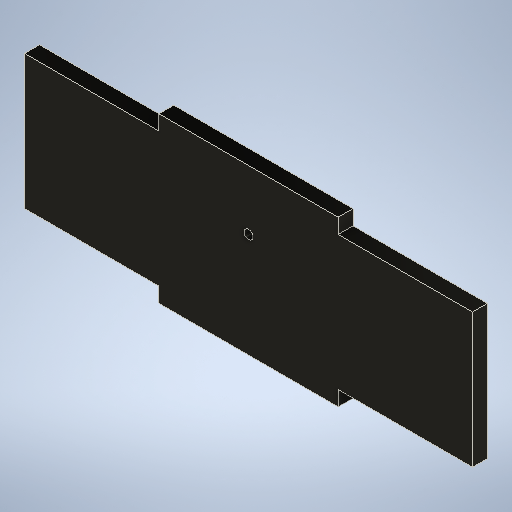
# Autodesk Inventor part: FRONT_1
Saved by Autodesk Inventor 2025.3 (Build 293356030, 356C)
## iProperties
Created: 2026-06-30
Part Number: FRONT_1
Material: ABS Plastic
Document SubType Name: Modeling
Designer: user
Density: 1.06 g/cm^3
Appearance: Gunmetal
Author: user
Autodesk Inventor part; units mm, degrees
ref_plane "YZ Plane" through (0, 0, 0) normal (1, 0, 0) x (0, 1, 0)
ref_plane "XZ Plane" through (0, 0, 0) normal (0, 1, 0) x (-1, 0, 0)
ref_plane "XY Plane" through (0, 0, 0) normal (0, 0, 1) x (1, 0, 0)
sketch "Sketch1" plane through (0, 0, 0) normal (0, 0, 1) x (1, 0, 0)
  line L0 (0, 0) -> (150, 0)
  line L1 (150, 0) -> (150, 45)
  line L2 (150, 45) -> (0, 45)
  line L3 (0, 45) -> (0, 0)
  line L4 (45, 0) -> (105, 0)
  line L5 (105, 0) -> (105, -5)
  line L6 (105, -5) -> (45, -5)
  line L7 (45, -5) -> (45, 0)
  line L8 (45, 45) -> (105, 45)
  line L9 (105, 45) -> (105, 50)
  line L10 (105, 50) -> (45, 50)
  line L11 (45, 50) -> (45, 45)
  point P0 (105, 45)
  dimension "d0" = 150
  dimension "d1" = 45
  dimension "d2" = 60
  dimension "d3" = 5
  dimension "d4" = 60
  dimension "d5" = 5
  dimension "d6" = 45
  dimension "d7" = 45
  constraints: 24 end point, 6 parallel, 3 horizontal, 3 perpendicular, 2 point on line
  measures "d0" distance of L2.end L1.end
  measures "d1" distance of L1.end L0.end
  measures "d2" distance of L5.end L6.end
  measures "d3" distance of L4.end L5.end
  measures "d4" distance of L10.end L9.end
  measures "d5" distance of L9.end L8.end
  measures "d6" distance between parallel lines of L3 L11
  measures "d7" distance between parallel lines of L7 L3
extrude "Extrusion1" add sketch "Sketch1" along normal blind 5
sketch "Sketch2" plane through (0, 0, 5) normal (0, 0, 1) x (1, 0, 0)
  line L0 (45, -5) -> (105, -5) projected
  line L1 (45, 50) -> (45, 45) projected
  line L2 (105, 50) -> (45, 50) projected
  point P0 (0, 0)
  point P1 (75, 30)
  dimension "d18" = 30
  dimension "d19" = 20
  measures "d18" distance from line of point (75, 30) L1
  measures "d19" distance from line of L2 point (75, 30)
hole "Hole1" at (75, 30, 5) direction (0, 0, -1) diameter 3 end through all
body "Solid1"
